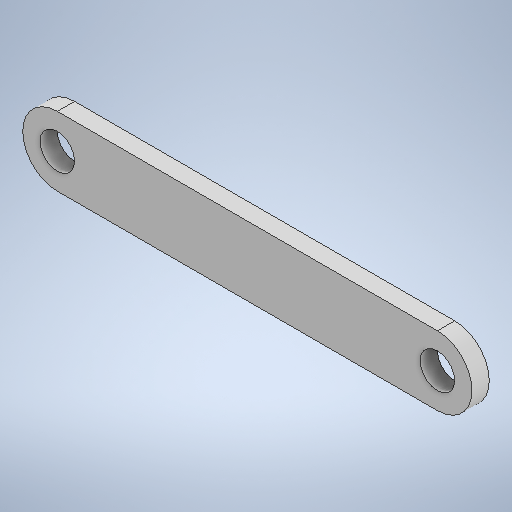
# Autodesk Inventor part: CS-Crank
Saved by Autodesk Inventor 2025.1 (Build 291241000, 241)
## iProperties
Created: 2025-04-02
Part Number: CS-Crank
Material: Generic
Document SubType Name: Modeling
Designer: a00584475
Density: 1 g/cm^3
Appearance: Default
Author: a00584475
Autodesk Inventor part; units mm, degrees
ref_plane "YZ Plane" through (0, 0, 0) normal (1, 0, 0) x (0, 1, 0)
ref_plane "XZ Plane" through (0, 0, 0) normal (0, 1, 0) x (-1, 0, 0)
ref_plane "XY Plane" through (0, 0, 0) normal (0, 0, 1) x (1, 0, 0)
sketch "Sketch1" plane through (0, 0, 0) normal (0, 0, 1) x (1, 0, 0)
  line L0 (-69.85, 0) -> (69.85, 0) construction
  line L1 (-69.85, -12.7) -> (69.85, -12.7)
  line L2 (69.85, 12.7) -> (-69.85, 12.7)
  arc A0 (-69.85, 12.7) -> (-69.85, -12.7) centre (-69.85, 0) ccw
  arc A1 (69.85, -12.7) -> (69.85, 12.7) centre (69.85, 0) ccw
  circle A2 centre (-69.85, 0) radius 6.35
  circle A3 centre (69.85, 0) radius 6.35
  point P0 (0, 0)
  dimension "d0" = 69.85
  dimension "d1" = 25.4
  dimension "d2" = 12.7
  dimension "d3" = 12.7
  constraints: 8 end point, 4 centre point, 4 point on circle, 4 tangent, 2 coincident, 1 horizontal, 1 midpoint, 1 parallel
  measures "d0" distance of point (0, 0) L0.end
  measures "d1" diameter of A1
  measures "d2" diameter of A2
  measures "d3" diameter of A3
extrude "Extrusion1" add sketch "Sketch1" along normal blind 6.35
body "Solid1"
